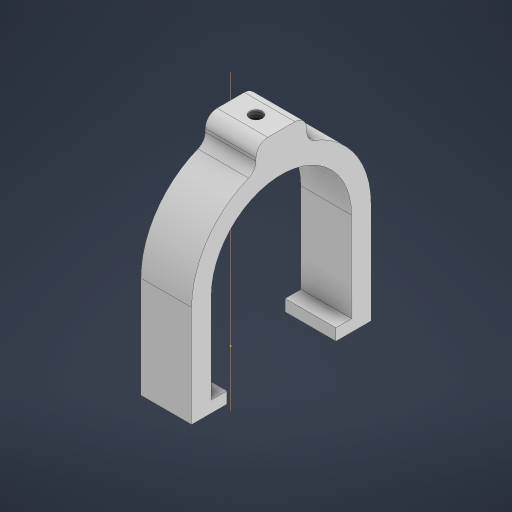
# Autodesk Inventor part: Część27
Saved by Autodesk Inventor 2023 (Build 270158000, 158)
## iProperties
Created: 2023-05-09
Part Number: Część27
Material: Ogólny
Document SubType Name: Modeling
Designer: Adam
Density: 1 g/cm^3
Appearance: Domyślna
Author: Adam
Autodesk Inventor part; units mm, degrees
ref_plane "YZ Plane" through (0, 0, 0) normal (1, 0, 0) x (0, 1, 0)
ref_plane "XZ Plane" through (0, 0, 0) normal (0, 1, 0) x (-1, 0, 0)
ref_plane "XY Plane" through (0, 0, 0) normal (0, 0, 1) x (1, 0, 0)
sketch "Szkic1" plane through (0, 0, 0) normal (1, 0, 0) x (0, 1, 0)
  line L0 (3.5782, 14) -> (0.5782, 14)
  line L1 (0.5782, 14) -> (0.5782, 23)
  line L2 (0.5782, 23) -> (26.5782, 23)
  arc A0 (49.5782, 0) -> (26.5782, 23) centre (26.5782, 0) ccw
  line L3 (3.5782, 14) -> (3.5782, 18)
  line L4 (3.5782, 18) -> (26.5782, 18)
  arc A1 (44.5782, 0) -> (26.5782, 18) centre (26.5782, 0) ccw
  line L5 (3.5782, -14) -> (0.5782, -14)
  line L6 (0.5782, -14) -> (0.5782, -23)
  line L7 (0.5782, -23) -> (26.5782, -23)
  arc A2 (26.5782, -23) -> (49.5782, 0) centre (26.5782, 0) ccw
  line L8 (3.5782, -14) -> (3.5782, -18)
  line L9 (3.5782, -18) -> (26.5782, -18)
  arc A3 (26.5782, -18) -> (44.5782, 0) centre (26.5782, 0) ccw
  line L10 (51.5782, 6.5) -> (44.5782, 6.5)
  line L11 (44.5782, 6.5) -> (44.5782, -6.5)
  line L12 (44.5782, -6.5) -> (51.5782, -6.5)
  line L13 (54.5782, -3.5) -> (54.5782, 3.5)
  arc A4 (54.5782, 3.5) -> (51.5782, 6.5) centre (51.5782, 3.5) ccw
  arc A5 (51.5782, -6.5) -> (54.5782, -3.5) centre (51.5782, -3.5) ccw
  point P0 (0, 0)
  point P1 (2.0782, 14)
  point P2 (3.5782, 16)
  point P3 (2.0782, -14)
  point P4 (0.5782, 18.5)
  point P5 (48.6406, -6.5)
  point P6 (48.6406, 6.5)
  dimension "d0" = 9
  dimension "d2" = 5
  dimension "d3" = 3
  dimension "d4" = 23
  dimension "d5" = 14
  dimension "d6" = 14
  dimension "d7" = 13
  dimension "d8" = 54
  dimension "d9" = 3
  dimension "d10" = 3
  constraints: 28 end point, 12 point on circle, 6 centre point, 4 midpoint, 4 perpendicular, 4 tangent, 2 coincident, 2 collinear, 2 horizontal, 2 parallel, 1 vertical
  measures "d0" distance from line of point (2.078, 14) L2
  measures "d2" distance between parallel lines of L4 L2
  measures "d3" distance from line of L1 point (3.578, 16)
  measures "d4" radius of A0
  measures "d5" vertical distance of point (2.078, -14) point (0, 0)
  measures "d6" vertical distance of point (0, 0) point (2.078, 14)
  measures "d7" distance of L11.end L10.end
  measures "d8" distance from line of point (0.578, 18.5) L13
  measures "d9" radius of A4
  measures "d10" radius of A5
sketch "Szkic2" plane through (0, 0, 0) normal (1, 0, 0) x (0, 1, 0)
  point P0 (0, 0)
extrude "Wyciągnięcie proste1" add sketch "Szkic1" along normal blind 13
fillet "Zaokrąglenie1" radius 3 1 edges at (6.5, 48.6406, -6.5)
fillet "Zaokrąglenie2" radius 3 1 edges at (6.5, 48.6406, 6.5)
sketch "Szkic3" plane through (0, 54.5782, 3.5) normal (0, 1, 0) x (1, 0, 0)
  point P0 (0, 3.5)
  point P1 (6.5, 3.5)
hole "Otwór1" at (6.5, 54.5782, 0) direction (0, -1, 0) diameter 3.242 end through all thread size "M4x0.7" class "6H" standard "ANSI Metric M Profile"
